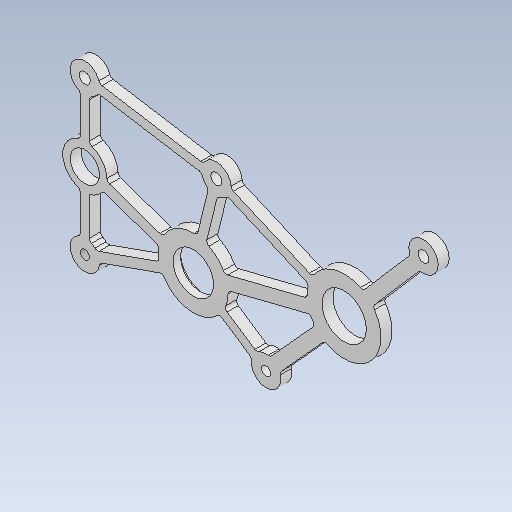
# Autodesk Inventor part: 脚ギアトレイン2
Saved by Autodesk Inventor 2020.2 (Build 242310000, 310)
## iProperties
Created: 2020-03-11
Part Number: 脚ギアトレイン2
Material: ポリカーボネート、スモーク
Document SubType Name: Modeling
Designer: aoyam
Density: 1.2 g/cm^3
Appearance: ポリカーボネート - スモーク
Mass: 8.50489 g
Surface Area: 44.6914 cm^2
Volume: 3.02665 cm^3
Author: aoyam
Autodesk Inventor part; units mm, degrees
ref_plane "YZ Plane" through (0, 0, 0) normal (1, 0, 0) x (0, 1, 0)
ref_plane "XZ Plane" through (0, 0, 0) normal (0, 1, 0) x (-1, 0, 0)
ref_plane "XY Plane" through (0, 0, 0) normal (0, 0, 1) x (1, 0, 0)
sketch "スケッチ1" plane through (0, 0, 0) normal (0, 0, 1) x (1, 0, 0)
  circle A0 centre (93.6, 0) radius 6.025
  circle A1 centre (93.6, 0) radius 8.025
  circle A2 centre (23.2, 0) radius 4
  circle A3 centre (23.2, 0) radius 14.1 construction
  circle A4 centre (93.6, 0) radius 25.1 construction
  circle A5 centre (23.2, 0) radius 16 construction
  circle A6 centre (93.6, 0) radius 27
  line L0 (93.6, 0) -> (43.9613, 30) construction
  line L1 (43.9613, 30) -> (43.9613, 0) construction
  line L2 (93.6, 0) -> (0, 0)
  circle A7 centre (43.9613, 30) radius 1.5
  circle A8 centre (52.6656, -10.2575) radius 5.5
  circle A9 centre (52.6656, -10.2575) radius 19 construction
  circle A10 centre (52.6656, -10.2575) radius 17.1 construction
  circle A11 centre (23.2, 20.8573) radius 1.5
  circle A12 centre (23.2, -20.6986) radius 1.25
  circle A13 centre (58.9094, 15) radius 1.5
  circle A14 centre (72.4024, -23.4155) radius 1.25
  circle A15 centre (115.1455, 24.8573) radius 1.5
  circle A16 centre (23.2, -20.6986) radius 4
  circle A17 centre (23.2, 20.8573) radius 4
  circle A18 centre (72.4024, -23.4155) radius 4
  circle A19 centre (58.9094, 15) radius 4 construction
  circle A20 centre (115.1455, 24.8573) radius 4
  line L3 (23.2, 20.8573) -> (23.2, 0) construction
  line L4 (21.95, 20.8573) -> (21.95, 0)
  line L5 (24.45, 0) -> (24.45, 20.8573)
  arc A21 (24.45, 20.8573) -> (21.95, 20.8573) centre (23.2, 20.8573) ccw
  arc A22 (21.95, 0) -> (24.45, 0) centre (23.2, 0) ccw
  line L6 (23.2, 0) -> (23.2, -20.6986) construction
  line L7 (21.95, 0) -> (21.95, -20.6986)
  line L8 (24.45, -20.6986) -> (24.45, 0)
  arc A23 (24.45, 0) -> (21.95, 0) centre (23.2, 0) ccw
  arc A24 (21.95, -20.6986) -> (24.45, -20.6986) centre (23.2, -20.6986) ccw
  line L9 (23.2, -20.6986) -> (52.6656, -10.2575) construction
  line L10 (23.6175, -21.8768) -> (53.0831, -11.4357)
  line L11 (52.2481, -9.0793) -> (22.7825, -19.5204)
  arc A25 (22.7825, -19.5204) -> (23.6175, -21.8768) centre (23.2, -20.6986) ccw
  arc A26 (53.0831, -11.4357) -> (52.2481, -9.0793) centre (52.6656, -10.2575) ccw
  line L12 (52.6656, -10.2575) -> (72.4024, -23.4155) construction
  line L13 (51.9722, -11.2976) -> (71.709, -24.4556)
  line L14 (73.0958, -22.3754) -> (53.359, -9.2175)
  arc A27 (53.359, -9.2175) -> (51.9722, -11.2976) centre (52.6656, -10.2575) ccw
  arc A28 (71.709, -24.4556) -> (73.0958, -22.3754) centre (72.4024, -23.4155) ccw
  line L15 (72.4024, -23.4155) -> (93.6, 0) construction
  line L16 (73.6997, -24.59) -> (94.8974, -1.1745)
  line L17 (92.3026, 1.1745) -> (71.105, -22.241)
  arc A29 (71.105, -22.241) -> (73.6997, -24.59) centre (72.4024, -23.4155) ccw
  arc A30 (94.8974, -1.1745) -> (92.3026, 1.1745) centre (93.6, 0) ccw
  line L18 (93.6, 0) -> (115.1455, 24.8573) construction
  line L19 (94.9224, -1.1462) -> (116.4679, 23.7111)
  line L20 (113.8231, 26.0035) -> (92.2776, 1.1462)
  arc A31 (92.2776, 1.1462) -> (94.9224, -1.1462) centre (93.6, 0) ccw
  arc A32 (116.4679, 23.7111) -> (113.8231, 26.0035) centre (115.1455, 24.8573) ccw
  line L21 (23.2, 20.8573) -> (58.9094, 15) construction
  line L22 (22.9977, 19.6238) -> (58.7071, 13.7665)
  line L23 (59.1117, 16.2335) -> (23.4023, 22.0908)
  arc A33 (23.4023, 22.0908) -> (22.9977, 19.6238) centre (23.2, 20.8573) ccw
  arc A34 (58.7071, 13.7665) -> (59.1117, 16.2335) centre (58.9094, 15) ccw
  line L24 (58.9094, 15) -> (52.6656, -10.2575) construction
  line L25 (57.6959, 15.3) -> (51.4522, -9.9576)
  line L26 (53.8791, -10.5575) -> (60.1229, 14.7)
  arc A35 (60.1229, 14.7) -> (57.6959, 15.3) centre (58.9094, 15) ccw
  arc A36 (51.4522, -9.9576) -> (53.8791, -10.5575) centre (52.6656, -10.2575) ccw
  line L27 (93.6, 0) -> (58.9094, 15) construction
  line L28 (94.0961, 1.1473) -> (59.4055, 16.1473)
  line L29 (58.4133, 13.8527) -> (93.1039, -1.1473)
  arc A37 (93.1039, -1.1473) -> (94.0961, 1.1473) centre (93.6, 0) ccw
  arc A38 (59.4055, 16.1473) -> (58.4133, 13.8527) centre (58.9094, 15) ccw
  circle A39 centre (93.6, 0) radius 5
  circle A40 centre (52.6656, -10.2575) radius 5 construction
  circle A41 centre (23.2, 0) radius 6
  circle A42 centre (52.6656, -10.2575) radius 9.4
  circle A43 centre (93.6, 0) radius 10
  circle A44 centre (23.2, 0) radius 4.6
  circle A45 centre (52.6656, -10.2575) radius 6.5
  circle A46 centre (23.2, 20.8573) radius 1.5
  line L30 (23.2, 0) -> (52.6656, -10.2575) construction
  line L31 (22.7068, -1.4166) -> (52.1725, -11.6741)
  line L32 (53.1588, -8.8409) -> (23.6932, 1.4166)
  arc A47 (23.6932, 1.4166) -> (22.7068, -1.4166) centre (23.2, 0) ccw
  arc A48 (52.1725, -11.6741) -> (53.1588, -8.8409) centre (52.6656, -10.2575) ccw
  line L33 (52.6656, -10.2575) -> (93.6, 0) construction
  line L34 (53.091, -11.955) -> (94.0254, -1.6975)
  line L35 (93.1746, 1.6975) -> (52.2403, -8.56)
  arc A49 (52.2403, -8.56) -> (53.091, -11.955) centre (52.6656, -10.2575) ccw
  arc A50 (94.0254, -1.6975) -> (93.1746, 1.6975) centre (93.6, 0) ccw
  circle A51 centre (58.9094, 15) radius 4
  circle A52 centre (93.6, 0) radius 26
  point P0 (52.6656, 10.2575)
  point P1 (23.2, 10.4286)
  point P2 (23.2, -10.3493)
  point P3 (37.9328, -15.4781)
  point P4 (62.534, -16.8365)
  point P5 (83.0012, -11.7078)
  point P6 (104.3728, 12.4286)
  point P7 (41.0547, 17.9286)
  point P8 (55.7875, 2.3712)
  point P9 (76.2547, 7.5)
  point P10 (44.3016, -14.5474)
  point P11 (59.724, -16.4655)
  point P12 (74.2557, -25.0933)
  point P13 (89.6412, -6.9806)
  point P14 (100.0521, 4.772)
  point P15 (97.4073, 7.0644)
  point P16 (86.8201, 4.2934)
  point P17 (59.4055, 16.1473)
  point P18 (23.4023, 22.0908)
  point P19 (21.95, 5.8683)
  point P20 (21.95, -5.8683)
  point P21 (24.45, -18.9295)
  point P22 (24.45, -5.8683)
  point P23 (24.45, 5.8683)
  point P24 (24.45, 19.3855)
  point P25 (57.371, 13.9856)
  point P26 (53.6879, -0.9133)
  point P27 (43.4666, -12.191)
  point P28 (87.0465, -4.6316)
  point P29 (71.7784, -21.4972)
  point P30 (61.1108, -14.3854)
  point P31 (56.1149, -1.5132)
  point P32 (59.7685, 13.2667)
  point P33 (85.8279, 1.9988)
  point P34 (85.695, -6.1246)
  point P35 (83.9972, 2.7903)
  point P36 (98.7263, 8.5861)
  point P37 (84.9894, 5.085)
  point P38 (101.3711, 6.2937)
  point P39 (88.2897, -8.4735)
  point P40 (87.6941, 1.1918)
  point P41 (90.4504, 0)
  point P42 (85.575, 0)
  point P43 (87.575, 0)
  point P44 (27.1519, 21.4758)
  point P45 (21.95, 17.0576)
  point P46 (112.5695, 19.2135)
  point P47 (109.9247, 21.5059)
  point P48 (69.3402, 11.8516)
  point P49 (68.348, 9.557)
  point P50 (74.2204, -18.7997)
  point P51 (76.8151, -21.1487)
  point P52 (37.9328, -5.1288)
  point P53 (73.1328, -5.1288)
  point P54 (88.6863, 3.4865)
  point P55 (70.6899, -23.7762)
  point P56 (61.1989, -6.3151)
  point P57 (62.0497, -9.7101)
  point P58 (84.475, -4.0907)
  point P59 (83.6242, -0.6957)
  point P60 (44.3951, -5.7901)
  point P61 (29.1797, -0.4933)
  point P62 (28.1934, -3.3266)
  point P63 (43.4088, -8.6233)
  point P64 (114.112, 20.9931)
  point P65 (111.4673, 23.2855)
  point P66 (68.5475, -22.3479)
  point P67 (76.1137, -21.9234)
  point P68 (73.519, -19.5745)
  point P69 (69.9342, -20.2677)
  point P70 (59.211, 11.0114)
  point P71 (61.9009, 12.3446)
  point P72 (54.9575, 14.3815)
  point P73 (56.7841, 11.6113)
  point P74 (55.3622, 16.8485)
  point P75 (58.2935, 16.3677)
  point P76 (60.1665, 15.8183)
  point P77 (62.8931, 14.6393)
  point P78 (26.364, -18.2513)
  point P79 (24.45, -16.8989)
  point P80 (27.199, -20.6077)
  point P81 (21.95, -16.8989)
  point P82 (67.0395, -4.8516)
  point P83 (67.8902, -8.2466)
  point P84 (74.893, -18.0568)
  point P85 (68.8623, -8.003)
  point P86 (69.2669, 9.1596)
  point P87 (68.0116, -4.608)
  point P88 (70.2591, 11.4543)
  point P89 (109.2683, 20.7486)
  point P90 (26.7472, 19.0087)
  point P91 (24.45, 17.0576)
  point P92 (27.1951, 0.1975)
  point P93 (27.8, -0.013)
  point P94 (27.8, 0)
  point P95 (19.2, 0)
  dimension "d0" = 12.05
  dimension "d1" = 16.05
  dimension "d2" = 8
  dimension "d3" = 28.2
  dimension "d4" = 50.2
  dimension "d5" = 32
  dimension "d6" = 54
  dimension "d7" = 58
  dimension "d8" = 30
  dimension "d9" = 3
  dimension "d10" = 3
  dimension "d11" = 2.5
  dimension "d12" = 3
  dimension "d13" = 2.5
  dimension "d15" = 3
  dimension "d16" = 8
  dimension "d17" = 8
  dimension "d18" = 8
  dimension "d19" = 11
  dimension "d20" = 34.2
  dimension "d21" = 38
  dimension "d22" = 8
  dimension "d23" = 8
  dimension "d24" = 2.5
  dimension "d25" = 2.5
  dimension "d26" = 2.5
  dimension "d27" = 2.5
  dimension "d28" = 3.5
  dimension "d29" = 3.5
  dimension "d30" = 2.5
  dimension "d31" = 2.5
  dimension "d32" = 2.5
  dimension "d33" = 10
  dimension "d34" = 10
  dimension "d39" = 20
  dimension "d40" = 0.6
  dimension "d46" = 3
  dimension "d51" = 3
  dimension "d52" = 3.5
  dimension "d53" = 8
  dimension "d54" = 1
  dimension "d56" = 1.4
  dimension "d57" = 1
  dimension "d58" = 2.9
  constraints: 94 end point, 53 centre point, 46 tangent, 44 point on circle, 18 coincident, 11 midpoint, 11 parallel, 5 concentric, 2 horizontal, 2 point on line, 2 vertical, 1 perpendicular, 1 symmetric about line, 8 other
  measures "d0" diameter of A0
  measures "d1" diameter of A1
  measures "d2" diameter of A2
  measures "d3" diameter of A3
  measures "d4" diameter of A4
  measures "d5" diameter of A5
  measures "d6" diameter of A6
  measures "d7" distance of L0.start L0.end
  measures "d8" distance of L0.end L1.end
  measures "d9" diameter of A7
  measures "d10" diameter of A11
  measures "d11" diameter of A12
  measures "d12" diameter of A13
  measures "d13" diameter of A14
  measures "d15" diameter of A15
  measures "d16" diameter of A16
  measures "d17" diameter of A17
  measures "d18" diameter of A18
  measures "d19" diameter of A8
  measures "d20" diameter of A10
  measures "d21" diameter of A9
  measures "d22" diameter of A19
  measures "d23" diameter of A20
  measures "d24" diameter of A22
  measures "d25" diameter of A24
  measures "d26" diameter of A26
  measures "d27" diameter of A28
  measures "d28" diameter of A30
  measures "d29" diameter of A32
  measures "d30" diameter of A34
  measures "d31" diameter of A36
  measures "d32" diameter of A38
  measures "d33" diameter of A39
  measures "d34" diameter of A40
  measures "d39" diameter of A43
  measures "d40" radial gap between concentric circles of A2 A44
  measures "d46" diameter of A46
  measures "d51" diameter of A48
  measures "d52" diameter of A50
  measures "d53" diameter of A51
  measures "d54" radial gap between concentric circles of A6 A52
  measures "d56" radial gap between concentric circles of A41 A44
  measures "d57" radial gap between concentric circles of A8 A45
  measures "d58" radial gap between concentric circles of A42 A45
extrude "押し出し1" add sketch "スケッチ1" along normal blind 3 contours A0 L19 A1 L16 | A0 L20 A1 L19 | L16 A1 L17 A0 | A0 L28 A1 L20 | L19 A43 L16 A1 | A1 L20 A43 L19 | L34 A1 L35 L2 A0 | L17 A1 L34 | L16 A43 L17 A1 | A0 L29 A1 L28 | A1 L28 A43 L20 | A43 L20 A52 L19 | L2 L35 A0 | L17 A43 L34 A1 | L34 A43 L35 A1 | L16 A52 L17 A43 | A0 L35 L2 A1 L29 | A1 L29 A43 L28 | A52 L20 A6 L19 | L35 A1 L2 | L35 A43 L2 A1 | L34 A52 L35 A43 | L16 A6 L17 A52 | A1 L2 A43 L29 | A43 L29 A52 L28 | A6 L20 A20 L19 | L34 A6 L35 A52 | L16 A18 L17 A6 | A52 L29 A6 L28 | L19 A32 L20 A20 | A20 L20 A32 L19 | L34 A42 L35 A6 | L16 A29 L13 A14 L14 L17 A18 | A18 L13 A29 L16 | A6 L29 A51 L28 | L17 L14 A18 | L34 A45 L35 A42 | A42 L14 A45 L34 | A51 L29 L26 A13 L28 | L28 A13 L23 A51 | L14 L17 A29 L13 A18 | A18 L13 A42 L14 | L14 A14 L13 A29 L17 | L35 A45 L26 A42 | L34 A8 L35 A45 | A45 L14 A8 L34 | A51 L26 L29 | L26 A42 L25 L2 | L2 L25 A51 L26 | A42 L13 A45 L14 | L26 A45 L25 A42 | L35 A8 L26 A45 | A45 L13 A8 L14 | A42 L10 A45 L13 | L29 A13 L26 | L26 A51 L25 L22 A13 L29 | A13 L25 L22 A51 L23 | A51 L22 A17 L23 | L26 A8 L25 A45 | L25 A45 L32 A42 | A45 L10 A8 L13 | A42 L11 A45 L10 | L10 A16 L11 A42 | A51 L22 L25 | A13 L22 L25 | L23 A11 L4 A17 | A17 L22 L5 A11 L23 | A41 L32 A44 L2 | L2 A44 L5 A41 | L25 A8 L32 A45 | L32 A45 L31 A42 | A42 L31 A41 L32 | A45 L11 A8 L10 | L10 A12 L8 L11 A16 | A16 L7 A12 L10 | A42 L31 A45 L11 | L4 A11 L22 L5 A17 | A17 L5 A41 L4 | A17 L5 L22 | A44 L32 L2 | L2 L32 A2 L5 A44 | L5 A44 L4 A41 | A41 L31 A44 L32 | L32 A8 L31 A45 | A45 L31 A8 L11 | L11 L8 A16 | L4 A44 L2 A41 | L22 A11 L5 | L32 A44 L31 A2 L2 | L2 A2 L32 | L5 A2 L4 A44 | A41 L8 A44 L31 | L7 A41 L8 A16 | A16 L8 L11 A12 L7 | L8 A12 L11 | L4 A2 L2 A44 | L2 A44 L7 A41 | A44 L8 A2 L31 | A41 L7 A44 L8 | L2 A2 L7 A44 | A44 L7 A2 L8
extrude "押し出し2" cut sketch "スケッチ1" along normal blind 1 contours L34 A8 L35 A45 | A45 L14 A8 L34 | L35 A8 L26 A45 | A45 L13 A8 L14 | L26 A8 L25 A45 | A45 L10 A8 L13 | L25 A8 L32 A45 | A45 L11 A8 L10 | L32 A8 L31 A45 | A45 L31 A8 L11
sketch "スケッチ2" plane through (0, 0, 3) normal (0, 0, 1) x (1, 0, 0)
  line L0 (27.199, -20.6077) -> (44.3016, -14.5474) projected
  arc A0 (44.3016, -14.5474) -> (59.724, -16.4655) centre (52.6656, -10.2575) ccw projected
  line L1 (59.724, -16.4655) -> (68.5475, -22.3479) projected
  line L2 (76.1137, -21.9234) -> (88.2897, -8.4735) projected
  arc A1 (88.2897, -8.4735) -> (101.3711, 6.2937) centre (93.6, 0) ccw projected
  line L3 (101.3711, 6.2937) -> (114.112, 20.9931) projected
  arc A2 (98.7263, 8.5861) -> (84.9894, 5.085) centre (93.6, 0) ccw projected
  line L4 (55.3622, 16.8485) -> (27.1519, 21.4758) projected
  line L5 (21.95, 17.0576) -> (21.95, 5.8683) projected
  arc A3 (21.95, 5.8683) -> (21.95, -5.8683) centre (23.2, 0) ccw projected
  line L6 (21.95, -5.8683) -> (21.95, -16.8989) projected
  line L7 (24.45, 5.8683) -> (24.45, 17.0576) projected
  line L8 (26.7472, 19.0087) -> (54.9575, 14.3815) projected
  line L9 (56.7841, 11.6113) -> (53.6879, -0.9133) projected
  arc A4 (53.6879, -0.9133) -> (44.3951, -5.7901) centre (52.6656, -10.2575) ccw projected
  line L10 (43.4666, -12.191) -> (26.364, -18.2513) projected
  line L11 (24.45, -16.8989) -> (24.45, -5.8683) projected
  arc A5 (29.1797, -0.4933) -> (24.45, 5.8683) centre (23.2, 0) ccw projected
  circle A6 centre (58.9094, 15) radius 1.5 projected
  circle A7 centre (72.4024, -23.4155) radius 1.25 projected
  circle A8 centre (115.1455, 24.8573) radius 1.5 projected
  circle A9 centre (23.2, -20.6986) radius 1.25 projected
  circle A10 centre (23.2, 0) radius 4 projected
  circle A11 centre (93.6, 0) radius 6.025 projected
  line L12 (56.1149, -1.5132) -> (59.211, 11.0114) projected
  arc A12 (83.9972, 2.7903) -> (83.6242, -0.6957) centre (93.6, 0) ccw projected
  line L13 (69.9342, -20.2677) -> (61.1108, -14.3854) projected
  arc A13 (61.1989, -6.3151) -> (56.1149, -1.5132) centre (52.6656, -10.2575) ccw projected
  arc A14 (27.1519, 21.4758) -> (21.95, 17.0576) centre (23.2, 20.8573) ccw projected
  line L14 (28.1934, -3.3266) -> (43.4088, -8.6233) projected
  arc A15 (43.4088, -8.6233) -> (43.4666, -12.191) centre (52.6656, -10.2575) ccw projected
  arc A16 (26.364, -18.2513) -> (24.45, -16.8989) centre (23.2, -20.6986) ccw projected
  arc A17 (24.45, -5.8683) -> (28.1934, -3.3266) centre (23.2, 0) ccw projected
  arc A18 (84.475, -4.0907) -> (85.695, -6.1246) centre (93.6, 0) ccw projected
  arc A19 (73.519, -19.5745) -> (69.9342, -20.2677) centre (72.4024, -23.4155) ccw projected
  arc A20 (61.1108, -14.3854) -> (62.0497, -9.7101) centre (52.6656, -10.2575) ccw projected
  arc A21 (59.211, 11.0114) -> (61.9009, 12.3446) centre (58.9094, 15) ccw projected
  arc A22 (54.9575, 14.3815) -> (56.7841, 11.6113) centre (58.9094, 15) ccw projected
  line L15 (44.3951, -5.7901) -> (29.1797, -0.4933) projected
  arc A23 (21.95, -16.8989) -> (27.199, -20.6077) centre (23.2, -20.6986) ccw projected
  arc A24 (68.5475, -22.3479) -> (76.1137, -21.9234) centre (72.4024, -23.4155) ccw projected
  arc A25 (114.112, 20.9931) -> (111.4673, 23.2855) centre (115.1455, 24.8573) ccw projected
  arc A26 (62.8931, 14.6393) -> (55.3622, 16.8485) centre (58.9094, 15) ccw projected
  line L16 (61.9009, 12.3446) -> (83.9972, 2.7903) projected
  line L17 (83.6242, -0.6957) -> (61.1989, -6.3151) projected
  line L18 (85.695, -6.1246) -> (73.519, -19.5745) projected
  line L19 (62.0497, -9.7101) -> (84.475, -4.0907) projected
  line L20 (111.4673, 23.2855) -> (98.7263, 8.5861) projected
  line L21 (84.9894, 5.085) -> (62.8931, 14.6393) projected
  arc A27 (24.45, 17.0576) -> (26.7472, 19.0087) centre (23.2, 20.8573) ccw projected
  point P0 (0, 0)
thread "ねじ1" size "M3x0.5" class "6H" standard "ANSI Metric M Profile" full length
fillet "フィレット1" radius 1.05 43 edges at (24.45, -16.8989, 1.5) (26.364, -18.2513, 1.5) (27.199, -20.6077, 1.5) (21.95, -16.8989, 1.5) (21.95, -5.8683, 1.5) (21.95, 17.0576, 1.5) (21.95, 5.8683, 1.5) (29.1797, -0.4933, 1.5) (24.45, 5.8683, 1.5) (28.1934, -3.3266, 1.5) (43.4088, -8.6233, 1.5) (43.4666, -12.191, 1.5) (44.3016, -14.5474, 1.5) (56.7841, 11.6113, 1.5) (54.9575, 14.3815, 1.5) (61.9009, 12.3446, 1.5) (59.724, -16.4655, 1.5) (59.211, 11.0114, 1.5) (56.1149, -1.5132, 1.5) (61.1989, -6.3151, 1.5) (44.3951, -5.7901, 1.5) (53.6879, -0.9133, 1.5) (55.3622, 16.8485, 1.5) (62.8931, 14.6393, 1.5) (62.0497, -9.7101, 1.5) (61.1108, -14.3854, 1.5) (73.519, -19.5745, 1.5) (69.9342, -20.2677, 1.5) (68.5475, -22.3479, 1.5) (76.1137, -21.9234, 1.5) (88.2897, -8.4735, 1.5) (101.3711, 6.2937, 1.5) (114.112, 20.9931, 1.5) (111.4673, 23.2855, 1.5) (84.9894, 5.085, 1.5) (98.7263, 8.5861, 1.5) (83.6242, -0.6957, 1.5) (83.9972, 2.7903, 1.5) (84.475, -4.0907, 1.5) (85.695, -6.1246, 1.5) (26.7472, 19.0087, 1.5) (24.45, 17.0576, 1.5) (27.1519, 21.4758, 1.5)
